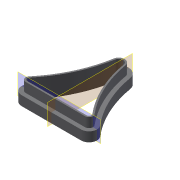
# Autodesk Inventor part: redefine
Saved by Autodesk Inventor 2022 Beta2 (Build 260130000, 130) ContinuousBuild 0
## iProperties
Shininess: 64.0
Length Units: 11269
Angle Units: 11279
Time Units: 11290
Mass Units: 11283
Length Display Precision: 3
Angle Display Precision: 2
Compacted: True
Part Number: redefine
Document SubType Name: Modeling
Created: 2004-04-15
Designer: mpaknia
Manufacturer: Standard
Standards Organization: Custom
Density: 1 g/cm^3
Material: Generic
Appearance: Light Gray
Density: 0.0
Volumn: 0.0
Area: 0.0
PropertySet Name: Model Information
Control State: 0
Master: False
Checked Out: False
Author: mpaknia
Autodesk Inventor part; units mm, degrees
ref_plane "XY Plane" through (0, 0, 0) normal (0, 0, 1) x (1, 0, 0)
sketch "Sketch1" plane through (0, 0, 0) normal (0, 0, 1) x (1, 0, 0)
  line L0 (0, 137.3747) -> (0, -23.9646) projected
  line L1 (-192.1248, 0) -> (256.1664, 0) projected
  arc A0 (-45.1628, 6.4251) -> (-37.5, -10) centre (-37.5, 0) ccw
  arc A1 (37.5, -10) -> (45.1628, 6.4251) centre (37.5, 0) ccw
  arc A2 (12.3157, 77.1386) -> (-12.3157, 77.1386) centre (0, 75) ccw
  arc A3 (-45.1628, 6.4251) -> (-12.3157, 77.1386) centre (-160.104, 102.802) ccw
  arc A4 (12.3157, 77.1386) -> (45.1628, 6.4251) centre (160.104, 102.802) ccw
  line L2 (-37.5, -10) -> (37.5, -10)
  dimension "d0" = 20
  dimension "d1" = 25
  dimension "d2" = 75
  dimension "d3" = 75
  dimension "d4" = 150
  constraints: 10 point on circle, 5 centre point, 5 tangent, 3 point on line, 2 end point, 2 equal radius, 1 horizontal alignment, 1 parallel, 1 other
  measures "d0" diameter of A0
  measures "d1" diameter of A2
  measures "d2" distance from line of L1 A2.centre
  measures "d3" distance of A1.centre A0.centre
  measures "d4" radius of A4
extrude "Extrusion1" add sketch "Sketch1" along normal blind 12
sketch "Sketch2" plane through (0, 0, 12) normal (0, 0, 1) x (1, 0, 0)
  arc A0 (-45.1628, 6.4251) -> (-12.3157, 77.1386) centre (-160.104, 102.802) ccw projected
  arc A1 (-45.1628, 6.4251) -> (-37.5, -10) centre (-37.5, 0) ccw projected
  line L0 (37.5, -10) -> (-37.5, -10) projected
  arc A2 (37.5, -10) -> (45.1628, 6.4251) centre (37.5, 0) ccw projected
  arc A3 (12.3157, 77.1386) -> (45.1628, 6.4251) centre (160.104, 102.802) ccw projected
  arc A4 (12.3157, 77.1386) -> (-12.3157, 77.1386) centre (0, 75) ccw projected
  arc A5 (-41.3314, 3.2126) -> (-7.3894, 76.2832) centre (-160.104, 102.802) ccw
  arc A6 (-41.3314, 3.2126) -> (-37.5, -5) centre (-37.5, 0) ccw
  line L1 (-37.5, -5) -> (37.5, -5)
  arc A7 (37.5, -5) -> (41.3314, 3.2126) centre (37.5, 0) ccw
  arc A8 (7.3894, 76.2832) -> (41.3314, 3.2126) centre (160.104, 102.802) ccw
  arc A9 (7.3894, 76.2832) -> (-7.3894, 76.2832) centre (0, 75) ccw
  dimension "d7" = 5
  constraints: 10 point on circle, 5 centre point, 2 end point, 5 other
  measures "d7" distance between parallel lines of L0 L1
extrude "Extrusion2" add sketch "Sketch2" along normal blind 12 contours A5 A9 A8 A7 L1 A6
sketch "Sketch3" plane through (0, 0, 24) normal (0, 0, 1) x (1, 0, 0)
  arc A0 (5.4189, 75.941) -> (-5.4189, 75.941) centre (0, 75) ccw
  arc A1 (5.4189, 75.941) -> (39.7988, 1.9275) centre (160.104, 102.802) ccw
  arc A2 (37.5, -3) -> (39.7988, 1.9275) centre (37.5, 0) ccw
  line L0 (37.5, -3) -> (-37.5, -3)
  arc A3 (-39.7988, 1.9275) -> (-37.5, -3) centre (-37.5, 0) ccw
  arc A4 (-39.7988, 1.9275) -> (-5.4189, 75.941) centre (-160.104, 102.802) ccw
  line L1 (0, 116.75) -> (0, -19.75) projected
  line L2 (-57, 0) -> (76, 0) projected
  dimension "d13" = 3
  constraints: 10 point on circle, 5 centre point, 5 tangent, 2 end point, 1 equal radius, 1 other
  measures "d13" radius of A3
extrude "Extrusion3" cut sketch "Sketch3" against normal through all
body "Solid1"
